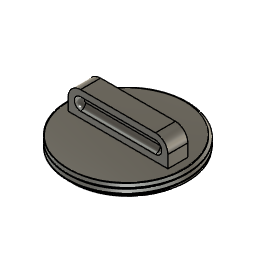
StampCase v6 (Autodesk Fusion 360 design; units mm, degrees)
Autodesk Fusion 360 part; units mm, degrees
sketch "Sketch1" plane through (0, 0, 0) normal (0, 0, 1) x (1, 0, 0)
  circle A0 centre (0, 0) radius 25
  dimension "d1" = 50
  constraint coincident A0.centre origin
  measures "d1" diameter of A0
extrude "Extrude1" add sketch "Sketch1" along normal blind 5
thread "Thread1" "ISO Metric profile 48.0 M48x2 6g" major diameter 47.822 minor diameter 45.524 pitch 2 angle 60 modelled right hand crest width 0.2789 on face at (24.9689, -1.2461, 3.3333) crest through (23.911, 0, -0.5)
sketch "Sketch2" plane through (0, 0, 5) normal (0, 0, 1) x (-1, 0, 0)
  spline S0 degree 3 poles (-10.1431, 21.653) (-12.9185, 20.274) (-15.3992, 18.3685) (-19.4686, 13.731) (-21.026, 11.0507) (-23.0119, 5.2684) (-23.4313, 2.2255) (-23.0765, -3.8221) (-22.3163, -6.7691) (-20.1341, -11.3095) (-19.0216, -13.0095) (-16.3874, -16.0631) (-14.8798, -17.4057) (-13.2155, -18.5327) knots 0 0 0 0 0.929748 0.929748 1.851289 1.851289 2.764621 2.764621 3.669742 3.669742 4.277081 4.277081 4.880618 4.880618 4.880618 4.880618
  arc A0 (-13.2155, -18.5327) -> (13.2155, -18.5327) centre (0, 0) ccw
  spline S1 degree 3 poles (13.2155, -18.5327) (15.6803, -16.8635) (17.7938, -14.7271) (21.1028, -9.7434) (22.2577, -6.9384) (23.4379, -1.0168) (23.4415, 2.0448) (22.2745, 8.026) (21.1048, 10.8859) (18.2751, 15.1852) (16.9027, 16.7677) (13.7706, 19.5421) (12.0224, 20.7193) (10.1431, 21.653) knots 0 0 0 0 0.893047 0.893047 1.794298 1.794298 2.703752 2.703752 3.621408 3.621408 4.246602 4.246602 4.875593 4.875593 4.875593 4.875593
  arc A1 (10.1431, 21.653) -> (-10.1431, 21.653) centre (0, 0) ccw
  line L0 (-20, 4) -> (20, 4)
  line L1 (20, 4) -> (20, -4)
  line L2 (20, -4) -> (-20, -4)
  line L3 (-20, -4) -> (-20, 4)
  line L4 (-20, 4) -> (20, -4) construction
  line L5 (20, 4) -> (-20, -4) construction
  constraint horizontal L0
  constraint perpendicular L0 L1
  constraint parallel L0 L2
  constraint parallel L1 L3
  constraint coincident L4 A0.centre
  constraint coincident L5 A0.centre
  constraint coincident A0.centre A1.centre
extrude "Extrude2" add sketch "Sketch2" along normal blind 10 contours L0 L1 L2 L3
fillet "Fillet1" radius 5 2 edges at (20, 0, 15) (-20, 0, 15)
sketch "Sketch3" plane through (0, -4, 0) normal (0, -1, 0) x (1, 0, 0)
  arc A0 (-15, 15) -> (-20, 10) centre (-15, 10) ccw
  line L0 (-20, 10) -> (-20, 5)
  line L1 (-20, 5) -> (20, 5)
  line L2 (20, 5) -> (20, 10)
  arc A1 (20, 10) -> (15, 15) centre (15, 10) ccw
  line L3 (15, 15) -> (-15, 15)
  line L4 (-15, 7.5) -> (15, 7.5)
  arc A2 (15, 7.5) -> (15, 12.5) centre (15, 10) ccw
  line L5 (15, 12.5) -> (-15, 12.5)
  arc A3 (-15, 12.5) -> (-15, 7.5) centre (-15, 10) ccw
  line L6 (-15, 10) -> (15, 10) construction
  point P0 (0, 10)
  dimension "d10" = 5
  constraint tangent L4 A2
  constraint tangent A2 L5
  constraint parallel L4 L5
  constraint tangent L5 A3
  constraint tangent L4 A3
  constraint coincident A1.centre A2.centre
  constraint horizontal L6
  constraint midpoint L6 P0
  measures "d10" diameter of A2
extrude "Extrude3" cut sketch "Sketch3" against normal blind 2 contours L4 A2 L5 A3
sketch "Sketch4" plane through (0, 4, 0) normal (0, 1, 0) x (-1, 0, 0)
  arc A0 (20, 10) -> (15, 15) centre (15, 10) ccw
  line L0 (15, 15) -> (-15, 15)
  arc A1 (-15, 15) -> (-20, 10) centre (-15, 10) ccw
  line L1 (-20, 10) -> (-20, 5)
  line L2 (-20, 5) -> (20, 5)
  line L3 (20, 5) -> (20, 10)
  line L4 (-15, 7.5) -> (15, 7.5)
  arc A2 (15, 7.5) -> (15, 12.5) centre (15, 10) ccw
  line L5 (15, 12.5) -> (-15, 12.5)
  arc A3 (-15, 12.5) -> (-15, 7.5) centre (-15, 10) ccw
  line L6 (-15, 10) -> (15, 10) construction
  point P0 (0, 10)
  dimension "d13" = 5
  constraint tangent L4 A2
  constraint tangent A2 L5
  constraint parallel L4 L5
  constraint tangent L5 A3
  constraint tangent L4 A3
  constraint coincident A0.centre A2.centre
  constraint midpoint L6 P0
  measures "d13" diameter of A2
extrude "Extrude4" cut sketch "Sketch4" against normal blind 2 contours L4 A2 L5 A3
fillet "Fillet2" radius 2 4 edges at (17.5, -2, 10) (0, -2, 7.5) (-17.5, -2, 10) (0, -2, 12.5)
fillet "Fillet3" radius 2 4 edges at (17.5, 2, 10) (0, 2, 12.5) (-17.5, 2, 10) (0, 2, 7.5)
sketch "Sketch5" plane through (0, 0, 0) normal (0, 0, -1) x (1, 0, 0)
  spline S0 degree 3 poles (-13.2155, 18.5327) (-15.6803, 16.8635) (-17.7938, 14.7271) (-21.1028, 9.7434) (-22.2577, 6.9384) (-23.4379, 1.0168) (-23.4415, -2.0448) (-22.2745, -8.026) (-21.1048, -10.8859) (-18.2751, -15.1852) (-16.9027, -16.7677) (-13.7706, -19.5421) (-12.0224, -20.7193) (-10.1431, -21.653) knots 0 0 0 0 0.893047 0.893047 1.794298 1.794298 2.703752 2.703752 3.621408 3.621408 4.246602 4.246602 4.875593 4.875593 4.875593 4.875593
  arc A0 (-10.1431, -21.653) -> (10.1431, -21.653) centre (0, 0) ccw
  spline S1 degree 3 poles (10.1431, -21.653) (12.9185, -20.274) (15.3992, -18.3685) (19.4686, -13.731) (21.026, -11.0507) (23.0119, -5.2684) (23.4313, -2.2255) (23.0765, 3.8221) (22.3163, 6.7691) (20.1341, 11.3095) (19.0216, 13.0095) (16.3874, 16.0631) (14.8798, 17.4057) (13.2155, 18.5327) knots 0 0 0 0 0.929748 0.929748 1.851289 1.851289 2.764621 2.764621 3.669742 3.669742 4.277081 4.277081 4.880618 4.880618 4.880618 4.880618
  arc A1 (13.2155, 18.5327) -> (-13.2155, 18.5327) centre (0, 0) ccw
  circle A2 centre (0, 0) radius 22.5
  dimension "d20" = 45
  constraint coincident A0.centre A1.centre
  measures "d20" diameter of A2
extrude "Extrude5" add sketch "Sketch5" along normal blind 0.6 contours A2
